# Autodesk Inventor part: Bottom Mold_RG
Saved by Autodesk Inventor 2016 (Build 200138000, 138)
## iProperties
Created: 2015-07-09
Part Number: Bottom Mold_RG
Material: Generic
Document SubType Name: Modeling
Designer: Samuel Clay
Density: 1 g/cm^3
Appearance: Default
Author: Samuel Clay
Autodesk Inventor part; units mm, degrees
ref_plane "YZ Plane" through (0, 0, 0) normal (1, 0, 0) x (0, 1, 0)
ref_plane "XZ Plane" through (0, 0, 0) normal (0, 1, 0) x (-1, 0, 0)
ref_plane "XY Plane" through (0, 0, 0) normal (0, 0, 1) x (1, 0, 0)
sketch "Sketch1" plane through (-0.0559, 0.5402, -2.54) normal (1, 0, 0) x (0, 1, 0)
  line L0 (-1.8712, 31.75) -> (1.8712, 31.75)
  arc A0 (-0.7615, -0.0266) -> (0.7615, -0.0266) centre (0, 0) ccw
  line L1 (-1.8712, 31.75) -> (-0.7615, -0.0266)
  line L2 (1.8712, 31.75) -> (0.7615, -0.0266)
  line L3 (0, 31.75) -> (0, -0.762)
  dimension "d0" = 0.762
  dimension "d1" = 31.75
  dimension "d2" = 88
  dimension "d3" = 88
  constraints: 8 end point, 3 point on circle, 2 tangent, 1 centre point, 1 coincident, 1 horizontal, 1 midpoint
  measures "d0" radius of A0
  measures "d1" distance from line of L0 A0.centre
  measures "d2" angle of L1 L0
  measures "d3" angle of L2 L0
revolve "Revolution1" add sketch "Sketch1" angle 360 about axis through (-0.0559, 0.5402, 29.21) along (0, 0, -1)
equation "\"d3\" = d2"
body "Solid1"
